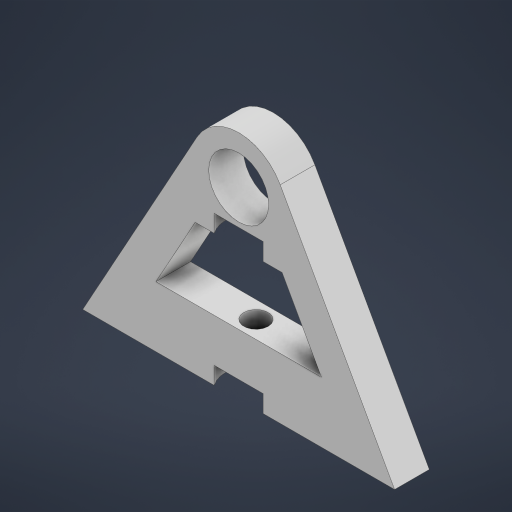
# Autodesk Inventor part: 96mmWheelBracket
Saved by Autodesk Inventor 2023 (Build 270158000, 158)
## iProperties
Created: 2022-10-27
Part Number: 96mmWheelBracket
Material: Generic
Document SubType Name: Modeling
Designer: Izack Waczko
Density: 1 g/cm^3
Appearance: Default
Author: Izack Waczko
## iProperties of the stored document 96mmWheelBracket_3DPrint.ipt
Part Number: 96mmWheelBracket_3DPrint
Material: Generic
Document SubType Name: Modeling
Designer: izack
Appearance: Default
Author: izack
Autodesk Inventor part; units mm, degrees
ref_plane "YZ Plane" through (0, 0, 0) normal (1, 0, 0) x (0, 1, 0)
ref_plane "XZ Plane" through (0, 0, 0) normal (0, 1, 0) x (-1, 0, 0)
ref_plane "XY Plane" through (0, 0, 0) normal (0, 0, 1) x (1, 0, 0)
sketch "Sketch1" plane through (0, 0, 0) normal (0, 0, 1) x (1, 0, 0)
  circle A0 centre (0, 0) radius 8.7
  arc A1 (11.985896, 6.635383) -> (-11.985896, 6.635383) centre (0, 0) ccw
  line L0 (0, 52.910691) -> (0, -52.910691) construction
  line L1 (-45, -53) -> (45, -53)
  line L2 (-45, -53) -> (-11.985896, 6.635383)
  line L3 (45, -53) -> (11.985896, 6.635383)
  line L4 (12.533127, -15) -> (23.881912, -35.5)
  line L5 (23.881912, -35.5) -> (-23.881912, -35.5)
  line L6 (-12.533127, -15) -> (12.533127, -15)
  line L7 (-23.881912, -35.5) -> (-12.533127, -15)
  circle A2 centre (0, 0) radius 8.65
  dimension "d0" = 5
  dimension "d1" = 53
  dimension "d2" = 90
  dimension "d3" = 45
  dimension "d12" = 17.5
  dimension "d13" = 15
  dimension "d15" = 10
  dimension "d16" = 10
  dimension "d41" = 17.3
  constraints: 16 end point, 2 centre point, 2 coincident, 2 horizontal, 2 parallel, 2 point on circle, 2 tangent, 1 midpoint, 1 vertical
  measures "d0" radial gap between concentric circles of A0 A1
  measures "d1" distance from line of L1 point (0, 0)
  measures "d2" distance of L1.start L1.end
  measures "d3" horizontal distance of point (0, 0) L1.end
  measures "d12" distance between parallel lines of L1 L5
  measures "d13" distance from line of L6 A0.centre
  measures "d15" distance between parallel lines of L2 L7
  measures "d16" distance between parallel lines of L3 L4
  measures "d41" diameter of A2
sketch "Sketch1 outline for Extrusion1" plane through (0, 0, 0) normal (0, 0, 1) x (1, 0, 0)
  line L0 (-45, -53) -> (45, -53)
  line L1 (45, -53) -> (11.985896, 6.635383)
  arc A0 (11.985896, 6.635383) -> (-11.985896, 6.635383) centre (0, 0) ccw
  line L2 (-11.985896, 6.635383) -> (-45, -53)
  line L3 (12.533127, -15) -> (23.881912, -35.5)
  line L4 (23.881912, -35.5) -> (-23.881912, -35.5)
  line L5 (-23.881912, -35.5) -> (-12.533127, -15)
  line L6 (-12.533127, -15) -> (12.533127, -15)
  circle A1 centre (0, 0) radius 8.65
extrude "Extrusion1" add sketch "Sketch1 outline for Extrusion1" along normal blind 5
sketch "Sketch2" plane through (0, 0, 5) normal (0, 0, 1) x (1, 0, 0)
  line L0 (45, -53) -> (11.985896, 6.635383)
  arc A0 (11.985896, 6.635383) -> (-11.985896, 6.635383) centre (0, 0) ccw
  line L1 (-11.985896, 6.635383) -> (-45, -53)
  line L2 (-45, -53) -> (45, -53)
  line L3 (12.533127, -15) -> (23.881912, -35.5)
  line L4 (23.881912, -35.5) -> (-23.881912, -35.5)
  line L5 (-23.881912, -35.5) -> (-12.533127, -15)
  line L6 (-12.533127, -15) -> (12.533127, -15)
  line L7 (39.910172, -50) -> (9.361247, 5.182379)
  arc A1 (9.361247, 5.182379) -> (-9.361247, 5.182379) centre (0, 0) ccw
  line L8 (-9.361247, 5.182379) -> (-39.910172, -50)
  line L9 (-39.910172, -50) -> (39.910172, -50)
  line L10 (-14.301359, -12) -> (-28.97174, -38.5)
  line L11 (-28.97174, -38.5) -> (28.97174, -38.5)
  line L12 (28.97174, -38.5) -> (14.301359, -12)
  line L13 (14.301359, -12) -> (-14.301359, -12)
  circle A2 centre (0, 0) radius 8.65
  point P0 (0, 0)
  point P1 (-11.653536, 1.041678)
  point P2 (11.653536, 1.041678)
  dimension "d19" = 3
  dimension "d20" = 3
  dimension "d42" = 17.3
  constraints: 14 end point, 2 centre point, 2 point on circle, 6 other
  measures "d19" distance between parallel lines of L2 L9
  measures "d20" distance between parallel lines of L5 L10
  measures "d42" diameter of A2
extrude "Extrusion2" add sketch "Sketch2" along normal blind 5 contours L2 L1 A0 L0 | L9 L8 A1 L7 | L13 L12 L11 L10
sketch "Sketch3" plane through (-45, -53, 0) normal (0, -1, 0) x (1, 0, 0)
  line L0 (45, 0) -> (45, 10) construction
  line L1 (32.466873, 10) -> (57.533127, 10) construction
  line L2 (0, 0) -> (0, 10) construction
  line L3 (0, 5) -> (90, 5) construction
  line L4 (90, 0) -> (90, 10) construction
  line L5 (33.3, 5) -> (56.7, 5) construction
  circle A0 centre (45, 5) radius 8.65
  circle A1 centre (45, 5) radius 3.5
  circle A2 centre (45, 5) radius 4.5
  circle A3 centre (77.5, 5) radius 1.7
  circle A4 centre (65, 5) radius 1.7
  circle A5 centre (12.5, 5) radius 1.7
  circle A6 centre (25, 5) radius 1.7
  point P0 (56.653536, 5)
  point P1 (33.346464, 5)
  dimension "d24" = 17.3
  dimension "d25" = 7
  dimension "d32" = 9
  dimension "d35" = 3.4
  dimension "d36" = 12.5
  dimension "d37" = 3.4
  dimension "d38" = 12.5
  constraints: 7 centre point, 4 end point, 4 midpoint, 2 coincident, 2 point on line, 2 symmetric about line, 2 other
  measures "d24" diameter of A0
  measures "d25" diameter of A1
  measures "d32" diameter of A2
  measures "d35" diameter of A3
  measures "d36" distance from line of L4 A3.centre
  measures "d37" diameter of A4
  measures "d38" distance of A3.centre A4.centre
extrude "Extrusion3" cut sketch "Sketch3" against normal blind 5 contours A0 | A2
extrude "Extrusion4" cut sketch "Sketch3" against normal blind 43 contours A1
extrude "Extrusion5" cut sketch "Sketch3" against normal up to surface (5 mm away) from surface at -38 contours A0 | A2
extrude "Extrusion6" cut sketch "Sketch3" against normal blind 6 from surface at -38 contours A1 | A2
extrude "Extrusion7" cut sketch "Sketch3" against normal blind 13 contours A3 | A4 | A5 | A6
body "Solid1"
